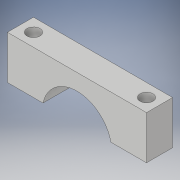
# Autodesk Inventor part: КВ33.044.208 - Зажим вакумной присоски
Saved by Autodesk Inventor 2019 (Build 230136000, 136)
## iProperties
Created: 2019-10-20
Part Number: КВ33.044.208 - Зажим вакумной присоски
Material: Типовые
Document SubType Name: Modeling
Designer: Петров Иван
Density: 1 g/cm^3
Appearance: По умолчанию
Author: Петров Иван
Autodesk Inventor part; units mm, degrees
ref_plane "YZ Plane" through (0, 0, 0) normal (1, 0, 0) x (0, 1, 0)
ref_plane "XZ Plane" through (0, 0, 0) normal (0, 1, 0) x (-1, 0, 0)
ref_plane "XY Plane" through (0, 0, 0) normal (0, 0, 1) x (1, 0, 0)
sketch "Эскиз1" plane through (0, 0, 0) normal (0, 1, 0) x (-1, 0, 0)
  line L0 (-4.0164, 1.5133) -> (-8.1434, 1.5133)
  circle A0 centre (-6.6434, 0.0133) radius 0.75
  line L1 (-4.0164, -1.4867) -> (-8.1434, -1.4867)
  line L2 (-4.0164, 1.5133) -> (-4.0164, -1.4867)
  line L3 (-4.0164, 1.5133) -> (-8.1434, 1.5133)
  line L4 (-8.1434, 1.5133) -> (-8.1434, -1.4867)
  circle A1 centre (6.3566, 0.0133) radius 0.75
  line L5 (3.7295, -1.4867) -> (3.7295, 1.5133)
  line L6 (7.8566, -1.4867) -> (3.7295, -1.4867)
  line L7 (7.8566, 1.5133) -> (7.8566, -1.4867)
  line L8 (3.7295, 1.5133) -> (7.8566, 1.5133)
  line L9 (-4.0164, 1.5133) -> (-4.0164, -1.4867)
  line L10 (3.7295, -1.4867) -> (-4.0164, -1.4867)
  line L11 (3.7295, -1.4867) -> (3.7295, 1.5133)
  line L12 (-4.0164, 1.5133) -> (3.7295, 1.5133)
  point P0 (0, 0)
  point P1 (0, 0)
  constraints: 26 end point, 2 centre point
extrude "Выдавливание1" add sketch "Эскиз1" along normal blind 5
sketch "Эскиз2" plane through (-7.8566, 0, 1.5133) normal (0, 0, 1) x (1, 0, 0)
  circle A0 centre (8, -0.857) radius 4
  line L0 (0, 0) -> (16, 0) projected
  dimension "d2" = 8
  dimension "d6" = 0.857
  dimension "d7" = 8
  constraints: 1 centre point
  measures "d2" diameter of A0
  measures "d6" distance from line of L0 A0.centre
  measures "d7" horizontal distance of L0.end A0.centre
extrude "Выдавливание2" cut sketch "Эскиз2" against normal through all
